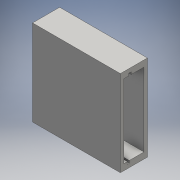
# Autodesk Inventor part: Plastic_Housing
Saved by Autodesk Inventor 2016 (Build 200138000, 138)
## iProperties
Created: 2018-07-17
Part Number: Plastic_Housing
Material: Generic
Document SubType Name: Modeling
Designer: Jorian Bruslind
Density: 1 g/cm^3
Appearance: Default
Author: Jorian Bruslind
Autodesk Inventor part; units mm, degrees
ref_plane "YZ Plane" through (0, 0, 0) normal (1, 0, 0) x (0, 1, 0)
ref_plane "XZ Plane" through (0, 0, 0) normal (0, 1, 0) x (-1, 0, 0)
ref_plane "XY Plane" through (0, 0, 0) normal (0, 0, 1) x (1, 0, 0)
sketch "Sketch1" plane through (0, 0, 0) normal (0, 1, 0) x (-1, 0, 0)
  line L0 (0, 0) -> (113.5, 0)
  line L1 (113.5, 0) -> (113.5, -111)
  line L2 (113.5, -111) -> (0, -111)
  line L3 (0, -111) -> (0, 0)
  dimension "d0" = 113.5
  dimension "d1" = 111
  constraints: 8 end point, 2 parallel, 1 horizontal, 1 perpendicular
  measures "d0" distance of L1.end L2.end
  measures "d1" distance of L0.end L1.end
extrude "Extrusion1" add sketch "Sketch1" along normal blind 35
sketch "Sketch2" plane through (0, 0, 0) normal (1, 0, 0) x (0, 0, -1)
  line L0 (0, 0) -> (0, 4.5)
  line L1 (0, 4.5) -> (8, 4.5)
  line L2 (8, 4.5) -> (103, 4.5)
  line L3 (103, 4.5) -> (103, 30.5)
  line L4 (103, 30.5) -> (8, 30.5)
  line L5 (8, 30.5) -> (8, 4.5)
  dimension "d4" = 4.5
  dimension "d5" = 8
  dimension "d6" = 95
  dimension "d7" = 26
  constraints: 12 end point, 2 horizontal, 2 parallel, 1 perpendicular, 1 vertical
  measures "d4" distance of L0.start L0.end
  measures "d5" distance of L0.end L1.end
  measures "d6" distance of L4.end L3.end
  measures "d7" distance of L3.end L2.end
extrude "Extrusion2" cut sketch "Sketch2" against normal blind 112
sketch "Sketch3" plane through (-112, 0, 0) normal (1, 0, 0) x (0, 0, -1)
  line L0 (8, 4.5) -> (8, 30.5) projected
  line L1 (8, 4.5) -> (44, 4.5)
  line L2 (103, 4.5) -> (8, 4.5) projected
  line L3 (8, 4.5) -> (8, 14.5)
  line L4 (8, 14.5) -> (44, 14.5)
  line L5 (44, 14.5) -> (44, 4.5)
  point P0 (0, 0)
  dimension "d10" = 36
  dimension "d11" = 10
  constraints: 8 end point, 2 perpendicular, 2 point on line
  measures "d10" distance of L0.start L1.end
  measures "d11" distance of L0.start L3.end
extrude "Extrusion3" add sketch "Sketch3" along normal blind 20
sketch "Sketch4" plane through (0, 0, 0) normal (1, 0, 0) x (0, 0, -1)
  line L0 (0, 0) -> (0, 7)
  line L1 (0, 7) -> (5, 7)
  line L2 (5, 7) -> (5, 14)
  line L3 (5, 14) -> (8, 14)
  line L4 (8, 4.5) -> (8, 30.5) projected
  line L5 (5, 7) -> (8, 7)
  line L6 (8, 14) -> (8, 7)
  line L7 (111, 0) -> (111, 6.5)
  line L8 (111, 6.5) -> (106, 6.5)
  line L9 (106, 6.5) -> (106, 11.5)
  line L10 (103, 30.5) -> (103, 4.5) projected
  line L11 (106, 6.5) -> (103, 6.5)
  line L12 (106, 11.5) -> (103, 11.5)
  line L13 (103, 6.5) -> (103, 11.5)
  line L14 (103, 6.5) -> (103, 9)
  line L15 (103, 30.5) -> (103, 4.5) projected
  line L16 (103, 9) -> (106, 9)
  line L17 (8, 7) -> (8, 10.5)
  line L18 (5, 10.5) -> (8, 10.5)
  dimension "d14" = 7
  dimension "d15" = 5
  dimension "d16" = 7
  dimension "d17" = 6.5
  dimension "d18" = 5
  dimension "d19" = 5
  constraints: 32 end point, 6 perpendicular, 6 point on line, 3 midpoint, 2 collinear, 2 horizontal, 2 vertical
  measures "d14" distance of L0.start L0.end
  measures "d15" distance of L0.end L1.end
  measures "d16" distance of L1.end L2.end
  measures "d17" distance of L7.start L7.end
  measures "d18" distance of L7.end L8.end
  measures "d19" distance of L8.end L9.end
extrude "Extrusion4" cut sketch "Sketch4" against normal blind 95 contours L2 L3 L4 L18 | L16 L10 L12 L9
body "Solid1"
